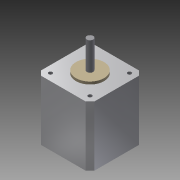
# Autodesk Inventor part: NEMA17StepperMotor
Saved by Autodesk Inventor 2014 SP1 (Build 180222100, 222)
## iProperties
Created: 2015-09-28
Part Number: NEMA17StepperMotor
Material: Generic
Document SubType Name: Modeling
Designer: Daniel Sikar
Density: 1 g/cm^3
Appearance: Default
Mass: 57.9466 g
Surface Area: 93.5788 cm^2
Volume: 57.9466 cm^3
Author: Daniel Sikar
Autodesk Inventor part; units mm, degrees
ref_plane "YZ Plane" through (0, 0, 0) normal (1, 0, 0) x (0, 1, 0)
ref_plane "XZ Plane" through (0, 0, 0) normal (0, 1, 0) x (-1, 0, 0)
ref_plane "XY Plane" through (0, 0, 0) normal (0, 0, 1) x (1, 0, 0)
sketch "Sketch1" plane through (0, 0, 0) normal (0, 0, 1) x (1, 0, 0)
  line L0 (0, 0) -> (42, 0)
  line L1 (42, 0) -> (42, 42)
  line L2 (42, 42) -> (0, 42)
  line L3 (0, 42) -> (0, 0)
  dimension "d0" = 42
  dimension "d1" = 42
  constraints: 8 end point, 2 parallel, 1 horizontal, 1 perpendicular
  measures "d0" distance of L2.end L1.end
  measures "d1" distance of L1.end L0.end
extrude "Extrusion1" add sketch "Sketch1" along normal blind 47
chamfer "Chamfer1" distance 3.5 angle 45 4 edges at (0, 42, 23.5) (0, 0, 23.5) (42, 0, 23.5) (42, 42, 23.5)
sketch "Sketch2" plane through (0, 0, 47) normal (0, 0, 1) x (1, 0, 0)
  circle A0 centre (21, 21) radius 11
  point P0 (0, 0)
  dimension "d7" = 22
  constraints: 1 centre point
  measures "d7" diameter of A0
extrude "Extrusion2" add sketch "Sketch2" along normal blind 2
sketch "Sketch3" plane through (21, 21, 49) normal (0, 0, 1) x (1, 0, 0)
  circle A0 centre (0, 0) radius 11 projected
  circle A1 centre (0, 0) radius 2.5
  point P0 (-21, -21)
  dimension "d10" = 5
  constraints: 1 centre point, 1 coincident
  measures "d10" diameter of A1
extrude "Extrusion3" add sketch "Sketch3" along normal blind 22 contours A1
sketch "Sketch4" plane through (0, 0, 47) normal (0, 0, 1) x (1, 0, 0)
  line L0 (0, 38.5) -> (0, 3.5) projected
  line L1 (3.5, 0) -> (38.5, 0) projected
  circle A0 centre (5.5, 36.5) radius 1.5
  circle A1 centre (36.5, 36.5) radius 1.5
  circle A2 centre (36.5, 5.5) radius 1.5
  circle A3 centre (5.5, 5.5) radius 1.5
  point P0 (0, 0)
  dimension "d13" = 3
  dimension "d14" = 3
  dimension "d15" = 3
  dimension "d16" = 3
  dimension "d17" = 31
  dimension "d18" = 31
  dimension "d19" = 31
  dimension "d20" = 31
  dimension "d21" = 5.5
  dimension "d22" = 5.5
  constraints: 4 centre point
  measures "d13" diameter of A0
  measures "d14" diameter of A1
  measures "d15" diameter of A2
  measures "d16" diameter of A3
  measures "d17" distance of A1.centre A0.centre
  measures "d18" distance of A2.centre A3.centre
  measures "d19" distance of A1.centre A2.centre
  measures "d20" distance of A3.centre A0.centre
  measures "d21" distance from line of A3.centre L0
  measures "d22" distance from line of L1 A3.centre
extrude "Extrusion4" cut sketch "Sketch4" against normal blind 4.5
body "Solid1"
